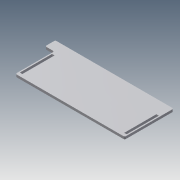
# Autodesk Inventor part: TopTopPanel
Saved by Autodesk Inventor 2014 (Build 180170000, 170)
## iProperties
Created: 2014-08-11
Part Number: TopTopPanel
Material: Generic
Document SubType Name: Modeling
Designer: Peele
Density: 1 g/cm^3
Appearance: White
Author: Peele
Autodesk Inventor part; units mm, degrees
ref_plane "YZ Plane" through (0, 0, 0) normal (1, 0, 0) x (0, 1, 0)
ref_plane "XZ Plane" through (0, 0, 0) normal (0, 1, 0) x (-1, 0, 0)
ref_plane "XY Plane" through (0, 0, 0) normal (0, 0, 1) x (1, 0, 0)
sketch "Sketch1" plane through (0, 0, 0) normal (0, 0, 1) x (1, 0, 0)
  line L0 (-134, -47.5) -> (134, -47.5)
  line L1 (134, -47.5) -> (134, 47.5)
  line L2 (134, 47.5) -> (-134, 47.5)
  line L3 (-134, 47.5) -> (-134, -47.5)
  line L4 (-134, -47.5) -> (134, 47.5) construction
  line L5 (134, -47.5) -> (-134, 47.5) construction
  point P0 (0, 0)
  dimension "d0" = 95
  dimension "d1" = 268
  constraints: 12 end point, 2 midpoint, 2 parallel, 1 horizontal, 1 perpendicular
  measures "d0" distance of L2.end L0.start
  measures "d1" distance of L0.start L0.end
extrude "Extrusion1" add sketch "Sketch1" along normal blind 6
sketch "Sketch2" plane through (0, 0, 6) normal (0, 0, 1) x (1, 0, 0)
  line L0 (-134, 47.5) -> (-134, -47.5) projected
  line L1 (-131.125, -39.5) -> (-124.875, -39.5)
  line L2 (-124.875, -39.5) -> (-124.875, 39.5)
  line L3 (-124.875, 39.5) -> (-131.125, 39.5)
  line L4 (-131.125, 39.5) -> (-131.125, -39.5)
  line L5 (-131.125, -39.5) -> (-124.875, 39.5) construction
  line L6 (-124.875, -39.5) -> (-131.125, 39.5) construction
  line L7 (124.875, -39.5) -> (131.125, -39.5)
  line L8 (131.125, -39.5) -> (131.125, 39.5)
  line L9 (131.125, 39.5) -> (124.875, 39.5)
  line L10 (124.875, 39.5) -> (124.875, -39.5)
  line L11 (124.875, -39.5) -> (131.125, 39.5) construction
  line L12 (131.125, -39.5) -> (124.875, 39.5) construction
  line L13 (-134, -47.5) -> (134, -47.5) projected
  line L14 (134, -47.5) -> (134, 47.5) projected
  point P0 (0, 0)
  point P1 (-128, 0)
  point P2 (128, 0)
  dimension "d4" = 6.25
  dimension "d5" = 2.875
  dimension "d23" = 8
  dimension "d24" = 2.875
  constraints: 24 end point, 4 midpoint, 4 parallel, 2 equal length, 2 horizontal, 2 horizontal alignment, 2 perpendicular
  measures "d4" distance of L2.end L3.end
  measures "d5" distance between parallel lines of L0 L4
  measures "d23" distance between parallel lines of L1 L13
  measures "d24" distance between parallel lines of L8 L14
extrude "Extrusion2" cut sketch "Sketch2" against normal through all
fillet "Fillet2" radius 3 2 edges at (-134, -47.5, 3) (134, -47.5, 3)
sketch "Sketch3" plane through (0, 0, 6) normal (0, 0, 1) x (1, 0, 0)
  line L0 (-131.125, -39.5) -> (-131.125, 39.5) projected
  line L1 (134, 47.5) -> (-134, 47.5) projected
  line L2 (-156.125, 47.5) -> (134, 47.5)
  line L3 (134, 47.5) -> (134, 72.5)
  line L4 (134, 72.5) -> (-156.125, 72.5)
  line L5 (-156.125, 72.5) -> (-156.125, 47.5)
  point P0 (0, 0)
  dimension "d12" = 25
  dimension "d13" = 25
  constraints: 8 end point, 2 parallel, 1 collinear, 1 horizontal, 1 perpendicular
  measures "d12" distance of L4.end L2.start
  measures "d13" distance between parallel lines of L5 L0
extrude "Extrusion3" add sketch "Sketch3" against normal blind 6
fillet "Fillet3" radius 3 4 edges at (134, 72.5, 3) (-156.125, 47.5, 3) (-156.125, 72.5, 3) (-134, 47.5, 3)
equation "\"d24\" = d5"
body "Solid1"
